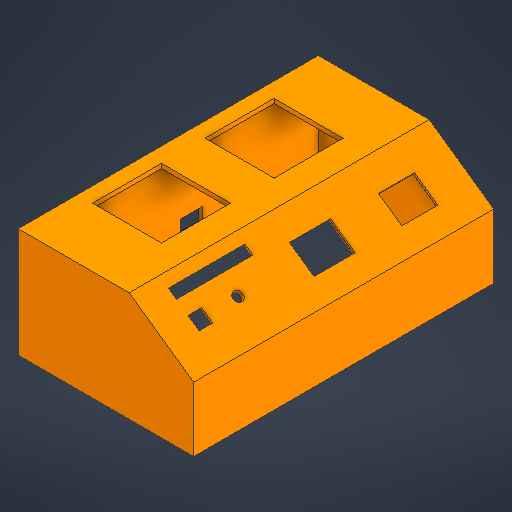
# Autodesk Inventor part: albox
Saved by Autodesk Inventor 2027 (Build 310192060, 192F)
## iProperties
Created: 2026-06-20
Part Number: albox
Material: Generic
Document SubType Name: Modeling
Designer: yunes
Density: 1 g/cm^3
Appearance: Default
Author: yunes
Autodesk Inventor part; units mm, degrees
ref_plane "YZ Plane" through (0, 0, 0) normal (1, 0, 0) x (0, 1, 0)
ref_plane "XZ Plane" through (0, 0, 0) normal (0, 1, 0) x (-1, 0, 0)
ref_plane "XY Plane" through (0, 0, 0) normal (0, 0, 1) x (1, 0, 0)
sketch "Sketch1" plane through (0, 0, 0) normal (0, 0, 1) x (1, 0, 0)
  line L0 (-60, 0) -> (-60, 70)
  line L1 (-60, 70) -> (10, 70)
  line L2 (10, 70) -> (50.9576, 41.3212)
  line L3 (50.9576, 41.3212) -> (50.9576, 0)
  line L4 (53.9576, 0) -> (53.9576, 42.8829)
  line L5 (53.9576, 42.8829) -> (10.9459, 73)
  line L6 (10.9459, 73) -> (-63, 73)
  line L7 (-63, 73) -> (-63, 0)
  line L8 (53.9576, 0) -> (50.9576, 0)
  line L9 (-60, 0) -> (-63, 0)
  point P0 (0, 0)
  dimension "d0" = 70
  dimension "d1" = 70
  dimension "d2" = 145
  dimension "d4" = 50
  dimension "d5" = 60
  dimension "d90" = 3
  constraints: 20 end point, 2 parallel, 2 perpendicular, 1 collinear, 1 horizontal, 1 horizontal alignment, 1 vertical, 3 other
  measures "d0" distance of L0.start L0.end
  measures "d1" distance of L0.end L1.end
  measures "d2" angle of L1 L2
  measures "d4" distance of L1.end L2.end
  measures "d5" distance from line of point (0, 0) L0
  measures "d90" distance between parallel lines of L3 L4
extrude "Extrusion1" add sketch "Sketch1" along normal blind 200
sketch "Sketch2" plane through (-63, 73, 0) normal (0, 1, 0) x (1, 0, 0)
  line L0 (10, -39.5) -> (56, -39.5)
  line L1 (56, -39.5) -> (56, -85.5)
  line L2 (56, -85.5) -> (10, -85.5)
  line L3 (10, -85.5) -> (10, -39.5)
  line L4 (0, 0) -> (0, -200) projected
  line L5 (73.9459, 0) -> (0, 0) projected
  line L6 (56, -160.5) -> (10, -160.5)
  line L7 (56, -114.5) -> (56, -160.5)
  line L8 (10, -160.5) -> (10, -114.5)
  line L9 (10, -114.5) -> (56, -114.5)
  point P0 (63, 0)
  dimension "d9" = 46
  dimension "d10" = 46
  dimension "d11" = 10
  dimension "d12" = 39.5
  dimension "d15" = 75
  constraints: 16 end point, 2 parallel, 1 horizontal, 1 perpendicular, 1 vertical, 8 other
  measures "d9" distance between parallel lines of L0 L2
  measures "d10" distance of L0.start L0.end
  measures "d11" distance between parallel lines of L4 L3
  measures "d12" distance between parallel lines of L5 L0
  measures "d15" distance of L1.end L6.start
extrude "Extrusion2" cut sketch "Sketch2" against normal blind 200
sketch "Sketch10" plane through (-63, 0, 0) normal (-1, 0, 0) x (0, 0, 1)
  line L0 (80, 27.5) -> (95, 27.5)
  line L1 (95, 27.5) -> (95, 17.5)
  line L2 (95, 17.5) -> (80, 17.5)
  line L3 (80, 17.5) -> (80, 27.5)
  line L4 (0, 0) -> (200, 0) projected
  line L5 (0, 73) -> (0, 0) projected
  dimension "d84" = 17.5
  dimension "d85" = 80
  dimension "d86" = 15
  dimension "d87" = 10
  constraints: 8 end point, 2 parallel, 1 horizontal, 1 perpendicular
  measures "d84" distance between parallel lines of L4 L2
  measures "d85" distance between parallel lines of L5 L3
  measures "d86" distance of L0.start L0.end
  measures "d87" distance of L0.end L1.end
extrude "Extrusion10" cut sketch "Sketch10" against normal blind 10
sketch "Sketch15" plane through (0, 0, 200) normal (0, 0, 1) x (1, 0, 0)
  line L0 (-60, 0) -> (-60, 70) projected
  line L1 (-60, 0) -> (-60, 70)
  line L2 (10, 70) -> (50.9576, 41.3212) projected
  line L3 (-60, 70) -> (10, 70)
  line L4 (50.9576, 41.3212) -> (50.9576, 0) projected
  line L5 (10, 70) -> (50.9576, 41.3212)
  line L6 (50.9576, 41.3212) -> (50.9576, 0)
  line L7 (50.9576, 0) -> (-60, 0)
  point P0 (0, 0)
  constraints: 10 end point, 2 perpendicular, 1 collinear, 1 vertical
extrude "Extrusion11" add sketch "Sketch15" against normal blind 3
pattern_linear "Rectangular Pattern3" count 2 spacing 197 along (0, 0, -1) of "Extrusion11"
sketch "Sketch16" plane through (10.9459, 73, 200) normal (0.5736, 0.8192, 0) x (0.8192, -0.5736, 0)
  line L0 (17.5076, 92.5) -> (37.5076, 92.5)
  line L1 (37.5076, 92.5) -> (37.5076, 120)
  line L2 (37.5076, 120) -> (17.5076, 120)
  line L3 (17.5076, 120) -> (17.5076, 92.5)
  line L4 (52.5076, 200) -> (52.5076, 0) projected
  line L5 (52.5076, 200) -> (0, 200) projected
  line L6 (18.5076, 151) -> (37.5076, 151)
  line L7 (37.5076, 151) -> (37.5076, 175)
  line L8 (37.5076, 175) -> (18.5076, 175)
  line L9 (18.5076, 175) -> (18.5076, 151)
  circle A0 centre (27.5076, 50) radius 3.25
  line L10 (23.5076, 20) -> (32.5076, 20)
  line L11 (32.5076, 20) -> (32.5076, 29)
  line L12 (32.5076, 29) -> (23.5076, 29)
  line L13 (23.5076, 29) -> (23.5076, 20)
  line L14 (52.5076, 0) -> (0, 0) projected
  line L15 (7.5, 20) -> (14, 20)
  line L16 (14, 20) -> (14, 71)
  line L17 (14, 71) -> (7.5, 71)
  line L18 (7.5, 71) -> (7.5, 20)
  line L19 (0, 200) -> (0, 0) projected
  point P0 (32.9047, 200)
  dimension "d99" = 20
  dimension "d100" = 27.5
  dimension "d101" = 15
  dimension "d102" = 80
  dimension "d103" = 24
  dimension "d104" = 19
  dimension "d105" = 15
  dimension "d106" = 25
  dimension "d107" = 6.5
  dimension "d108" = 9
  dimension "d109" = 9
  dimension "d110" = 20
  dimension "d111" = 25
  dimension "d112" = 50
  dimension "d113" = 20
  dimension "d114" = 6.5
  dimension "d115" = 51
  dimension "d116" = 7.5
  dimension "d117" = 20
  constraints: 32 end point, 8 parallel, 4 horizontal, 4 perpendicular, 1 centre point
  measures "d99" distance of L1.end L2.end
  measures "d100" distance of L2.end L0.start
  measures "d101" distance between parallel lines of L4 L1
  measures "d102" distance between parallel lines of L5 L2
  measures "d103" distance of L8.end L6.start
  measures "d104" distance of L6.start L6.end
  measures "d105" distance between parallel lines of L4 L7
  measures "d106" distance between parallel lines of L5 L8
  measures "d107" diameter of A0
  measures "d108" distance of L10.start L10.end
  measures "d109" distance of L12.end L10.start
  measures "d110" distance between parallel lines of L4 L11
  measures "d111" distance from line of L4 A0.centre
  measures "d112" distance from line of L14 A0.centre
  measures "d113" distance between parallel lines of L14 L10
  measures "d114" distance of L15.start L15.end
  measures "d115" distance of L17.end L15.start
  measures "d116" distance between parallel lines of L19 L18
  measures "d117" distance between parallel lines of L14 L15
extrude "Extrusion12" cut sketch "Sketch16" against normal blind 3 contours L3 L2 L1 L0 | L9 L8 L7 L6 | A0 | L13 L12 L11 L10 | L18 L17 L16 L15
sketch "Sketch17" plane through (50.9576, 41.3212, 3) normal (-0.5736, -0.8192, 0) x (0.8192, -0.5736, 0)
  line L0 (-38.4383, 76.75) -> (-8.4383, 76.75)
  line L1 (-8.4383, 76.75) -> (-8.4383, 104.75)
  line L2 (-8.4383, 104.75) -> (-38.4383, 104.75)
  line L3 (-38.4383, 104.75) -> (-38.4383, 76.75)
  line L4 (-46.1959, 118.5) -> (-34.1959, 118.5)
  line L5 (-34.1959, 118.5) -> (-34.1959, 184.5)
  line L6 (-34.1959, 184.5) -> (-46.1959, 184.5)
  line L7 (-46.1959, 184.5) -> (-46.1959, 118.5)
  line L8 (-29.4383, 166) -> (-16.4383, 166)
  line L9 (-16.4383, 166) -> (-16.4383, 179)
  line L10 (-16.4383, 179) -> (-29.4383, 179)
  line L11 (-29.4383, 179) -> (-29.4383, 166)
  line L12 (-36.9459, 177) -> (-36.9459, 126) projected
  line L13 (-43.4459, 177) -> (-36.9459, 177) projected
  line L14 (-27.4383, 177) -> (-18.4383, 177) projected
  line L15 (-27.4383, 168) -> (-27.4383, 177) projected
  line L16 (-33.4383, 104.5) -> (-13.4383, 104.5) projected
  line L17 (-33.4383, 77) -> (-33.4383, 104.5) projected
  line L18 (-35.4383, 21) -> (-10.4383, 21)
  line L19 (-10.4383, 21) -> (-10.4383, 47)
  line L20 (-10.4383, 47) -> (-35.4383, 47)
  line L21 (-35.4383, 47) -> (-35.4383, 21)
  line L22 (-32.4383, 46) -> (-13.4383, 46) projected
  line L23 (-32.4383, 22) -> (-32.4383, 46) projected
  point P0 (-18.0412, -3)
  point P1 (-34.1959, 151.5)
  point P2 (-36.9459, 151.5)
  point P3 (-40.1959, 177)
  point P4 (-40.1959, 184.5)
  point P5 (-22.9383, 179)
  point P6 (-22.9383, 177)
  point P7 (-29.4383, 172.5)
  point P8 (-27.4383, 172.5)
  point P9 (-23.4383, 104.75)
  point P10 (-23.4383, 104.5)
  point P11 (-33.4383, 90.75)
  point P12 (-38.4383, 90.75)
  point P13 (-22.9383, 47)
  point P14 (-22.9383, 46)
  point P15 (-32.4383, 34)
  point P16 (-35.4383, 34)
  dimension "d120" = 66
  dimension "d121" = 12
  dimension "d122" = 13
  dimension "d123" = 13
  dimension "d124" = 30
  dimension "d125" = 28
  dimension "d126" = 26
  dimension "d127" = 25
  constraints: 32 end point, 16 midpoint, 8 parallel, 4 horizontal, 4 horizontal alignment, 4 perpendicular, 4 vertical alignment
  measures "d120" distance of L6.end L4.start
  measures "d121" distance of L5.end L6.end
  measures "d122" distance of L9.end L10.end
  measures "d123" distance of L8.end L9.end
  measures "d124" distance of L1.end L2.end
  measures "d125" distance of L2.end L0.start
  measures "d126" distance of L20.end L18.start
  measures "d127" distance of L19.end L20.end
extrude "Extrusion13" cut sketch "Sketch17" against normal blind 1.5
body "Solid1"
